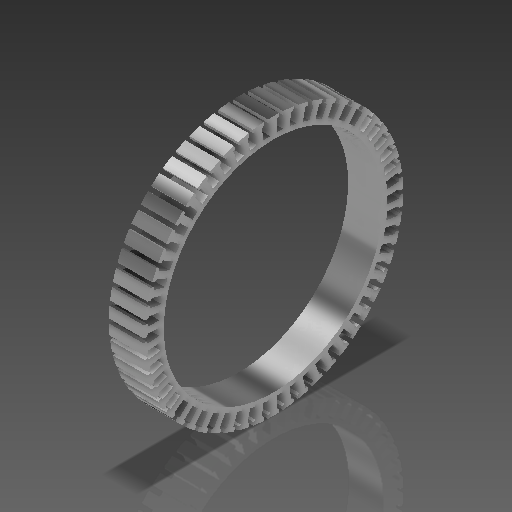
# Autodesk Inventor part: stator
Saved by Autodesk Inventor 2026.2 (Build 302298000, 298)
## iProperties
Created: 2026-05-19
Part Number: stator
Material: Generic
Document SubType Name: Modeling
Designer: LENOVO
Density: 1 g/cm^3
Appearance: Default
Author: LENOVO
Autodesk Inventor part; units mm, degrees
ref_plane "YZ Plane" through (0, 0, 0) normal (1, 0, 0) x (0, 1, 0)
ref_plane "XZ Plane" through (0, 0, 0) normal (0, 1, 0) x (-1, 0, 0)
ref_plane "XY Plane" through (0, 0, 0) normal (0, 0, 1) x (1, 0, 0)
sketch "Sketch1" plane through (0, 0, 0) normal (1, 0, 0) x (0, 1, 0)
  circle A0 centre (0, 0) radius 107.25
  line L0 (127, 0) -> (0, 0) construction
  line L1 (0, 0) -> (127, 0) construction
  line L2 (111.657, -3.1) -> (122.8894, -3.1)
  line L3 (123.8894, -5.3) -> (126.8894, -5.3) construction
  line L4 (123.8894, -5.3) -> (126.8894, -5.3)
  line L5 (111.657, 3.1) -> (122.8894, 3.1)
  line L6 (123.8894, 5.3) -> (126.8894, 5.3) construction
  line L7 (123.8894, 5.3) -> (126.8894, 5.3)
  line L8 (126.8894, -5.3) -> (123.8894, -5.3)
  line L9 (123.8894, -5.3) -> (122.8894, -3.1)
  line L10 (123.8894, 5.3) -> (122.8894, 3.1)
  line L11 (123.667, 9.1185) -> (126.6467, 9.4668) construction
  line L12 (123.667, 9.1185) -> (126.6467, 9.4668)
  line L13 (122.4364, 19.6468) -> (125.4161, 19.9951) construction
  line L14 (122.4364, 19.6468) -> (125.4161, 19.9951)
  line L15 (126.6467, 9.4668) -> (123.667, 9.1185)
  line L16 (123.667, 9.1185) -> (122.4183, 11.1875)
  line L17 (122.4364, 19.6468) -> (121.6985, 17.3456)
  line L18 (111.2619, 9.8835) -> (122.4183, 11.1875)
  line L19 (110.5421, 16.0416) -> (121.6985, 17.3456)
  line L20 (121.7722, 23.4137) -> (124.6913, 24.1056) construction
  line L21 (121.7722, 23.4137) -> (124.6913, 24.1056)
  line L22 (119.3276, 33.728) -> (122.2468, 34.4198) construction
  line L23 (119.3276, 33.728) -> (122.2468, 34.4198)
  line L24 (124.6913, 24.1056) -> (121.7722, 23.4137)
  line L25 (121.7722, 23.4137) -> (120.2918, 25.3238)
  line L26 (119.3276, 33.728) -> (118.862, 31.3567)
  line L27 (109.3622, 22.7334) -> (120.2918, 25.3238)
  line L28 (107.9323, 28.7663) -> (118.862, 31.3567)
  line L29 (118.2306, 37.3923) -> (121.0497, 38.4183) construction
  line L30 (118.2306, 37.3923) -> (121.0497, 38.4183)
  line L31 (114.6052, 47.353) -> (117.4243, 48.3791) construction
  line L32 (114.6052, 47.353) -> (117.4243, 48.3791)
  line L33 (121.0497, 38.4183) -> (118.2306, 37.3923)
  line L34 (118.2306, 37.3923) -> (116.5385, 39.1176)
  line L35 (114.6052, 47.353) -> (114.418, 44.9437)
  line L36 (105.9835, 35.2759) -> (116.5385, 39.1176)
  line L37 (103.863, 41.102) -> (114.418, 44.9437)
  line L38 (113.0902, 50.8652) -> (115.7711, 52.2116) construction
  line L39 (113.0902, 50.8652) -> (115.7711, 52.2116)
  line L40 (108.3329, 60.3377) -> (111.0138, 61.6841) construction
  line L41 (108.3329, 60.3377) -> (111.0138, 61.6841)
  line L42 (115.7711, 52.2116) -> (113.0902, 50.8652)
  line L43 (113.0902, 50.8652) -> (111.2092, 52.3824)
  line L44 (108.3329, 60.3377) -> (108.4267, 57.9229)
  line L45 (101.1716, 47.3413) -> (111.2092, 52.3824)
  line L46 (98.389, 52.8818) -> (108.4267, 57.9229)
  arc A1 (111.657, 3.1) -> (111.2619, 9.8835) centre (0, 0) ccw
  arc A2 (111.2619, -9.8835) -> (111.657, -3.1) centre (0, 0) ccw
  arc A3 (109.3622, -22.7334) -> (110.5421, -16.0416) centre (0, 0) ccw
  arc A4 (105.9835, -35.2759) -> (107.9323, -28.7663) centre (0, 0) ccw
  arc A5 (101.1716, -47.3413) -> (103.863, -41.102) centre (0, 0) ccw
  arc A6 (94.9915, -58.7665) -> (98.389, -52.8818) centre (0, 0) ccw
  arc A7 (87.5268, -69.397) -> (91.5846, -63.9465) centre (0, 0) ccw
  arc A8 (78.8785, -79.089) -> (83.5416, -74.1465) centre (0, 0) ccw
  arc A9 (69.1635, -87.7115) -> (74.3688, -83.3437) centre (0, 0) ccw
  arc A10 (58.5132, -95.1478) -> (64.1903, -91.4138) centre (0, 0) ccw
  arc A11 (47.0715, -101.2974) -> (53.1438, -98.2478) centre (0, 0) ccw
  arc A12 (34.9933, -106.0771) -> (41.3786, -103.7531) centre (0, 0) ccw
  arc A13 (22.4419, -109.4223) -> (29.0538, -107.8553) centre (0, 0) ccw
  arc A14 (9.587, -111.2878) -> (16.3361, -110.499) centre (0, 0) ccw
  arc A15 (-3.3975, -111.6483) -> (3.3975, -111.6483) centre (0, 0) ccw
  arc A16 (-16.3361, -110.499) -> (-9.587, -111.2878) centre (0, 0) ccw
  arc A17 (-29.0538, -107.8553) -> (-22.4419, -109.4223) centre (0, 0) ccw
  arc A18 (-41.3786, -103.7531) -> (-34.9933, -106.0771) centre (0, 0) ccw
  arc A19 (-53.1438, -98.2478) -> (-47.0715, -101.2974) centre (0, 0) ccw
  arc A20 (-64.1903, -91.4138) -> (-58.5132, -95.1478) centre (0, 0) ccw
  arc A21 (-74.3688, -83.3437) -> (-69.1635, -87.7115) centre (0, 0) ccw
  arc A22 (-83.5416, -74.1465) -> (-78.8785, -79.089) centre (0, 0) ccw
  arc A23 (-91.5846, -63.9465) -> (-87.5268, -69.397) centre (0, 0) ccw
  arc A24 (-98.389, -52.8818) -> (-94.9915, -58.7665) centre (0, 0) ccw
  arc A25 (-103.863, -41.102) -> (-101.1716, -47.3413) centre (0, 0) ccw
  arc A26 (-107.9323, -28.7663) -> (-105.9835, -35.2759) centre (0, 0) ccw
  arc A27 (-110.5421, -16.0416) -> (-109.3622, -22.7334) centre (0, 0) ccw
  arc A28 (-111.657, -3.1) -> (-111.2619, -9.8835) centre (0, 0) ccw
  arc A29 (-111.2619, 9.8835) -> (-111.657, 3.1) centre (0, 0) ccw
  arc A30 (-109.3622, 22.7334) -> (-110.5421, 16.0416) centre (0, 0) ccw
  arc A31 (-105.9835, 35.2759) -> (-107.9323, 28.7663) centre (0, 0) ccw
  arc A32 (-101.1716, 47.3413) -> (-103.863, 41.102) centre (0, 0) ccw
  arc A33 (-94.9915, 58.7665) -> (-98.389, 52.8818) centre (0, 0) ccw
  arc A34 (-87.5268, 69.397) -> (-91.5846, 63.9465) centre (0, 0) ccw
  arc A35 (-78.8785, 79.089) -> (-83.5416, 74.1465) centre (0, 0) ccw
  arc A36 (-69.1635, 87.7115) -> (-74.3688, 83.3437) centre (0, 0) ccw
  arc A37 (-58.5132, 95.1478) -> (-64.1903, 91.4138) centre (0, 0) ccw
  arc A38 (-47.0715, 101.2974) -> (-53.1438, 98.2478) centre (0, 0) ccw
  arc A39 (-34.9933, 106.0771) -> (-41.3786, 103.7531) centre (0, 0) ccw
  arc A40 (-22.4419, 109.4223) -> (-29.0538, 107.8553) centre (0, 0) ccw
  arc A41 (-9.587, 111.2878) -> (-16.3361, 110.499) centre (0, 0) ccw
  arc A42 (3.3975, 111.6483) -> (-3.3975, 111.6483) centre (0, 0) ccw
  arc A43 (16.3361, 110.499) -> (9.587, 111.2878) centre (0, 0) ccw
  arc A44 (29.0538, 107.8553) -> (22.4419, 109.4223) centre (0, 0) ccw
  arc A45 (41.3786, 103.7531) -> (34.9933, 106.0771) centre (0, 0) ccw
  arc A46 (53.1438, 98.2478) -> (47.0715, 101.2974) centre (0, 0) ccw
  arc A47 (64.1903, 91.4138) -> (58.5132, 95.1478) centre (0, 0) ccw
  arc A48 (74.3688, 83.3437) -> (69.1635, 87.7115) centre (0, 0) ccw
  arc A49 (83.5416, 74.1465) -> (78.8785, 79.089) centre (0, 0) ccw
  arc A50 (91.5846, 63.9465) -> (87.5268, 69.397) centre (0, 0) ccw
  arc A51 (98.389, 52.8818) -> (94.9915, 58.7665) centre (0, 0) ccw
  arc A52 (107.9323, 28.7663) -> (105.9835, 35.2759) centre (0, 0) ccw
  arc A53 (103.863, 41.102) -> (101.1716, 47.3413) centre (0, 0) ccw
  arc A54 (124.6913, 24.1056) -> (122.2468, 34.4198) centre (0, 0) ccw
  arc A55 (121.0497, 38.4183) -> (117.4243, 48.3791) centre (0, 0) ccw
  arc A56 (115.7711, 52.2116) -> (111.0138, 61.6841) centre (0, 0) ccw
  arc A57 (108.9269, 65.2988) -> (103.1021, 74.1549) centre (0, 0) ccw
  arc A58 (100.6097, 77.5029) -> (93.7961, 85.6229) centre (0, 0) ccw
  arc A59 (90.9318, 88.6589) -> (83.2217, 95.9331) centre (0, 0) ccw
  arc A60 (80.0243, 98.616) -> (71.5218, 104.9458) centre (0, 0) ccw
  arc A61 (68.0346, 107.2394) -> (58.8547, 112.5394) centre (0, 0) ccw
  arc A62 (55.1249, 114.4126) -> (45.3918, 118.6111) centre (0, 0) ccw
  arc A63 (41.4696, 120.0386) -> (31.3149, 123.0787) centre (0, 0) ccw
  arc A64 (27.2536, 124.0413) -> (16.8146, 125.882) centre (0, 0) ccw
  arc A65 (12.669, 126.3665) -> (2.0869, 126.9829) centre (0, 0) ccw
  arc A66 (-2.0869, 126.9829) -> (-12.669, 126.3665) centre (0, 0) ccw
  arc A67 (-16.8146, 125.882) -> (-27.2536, 124.0413) centre (0, 0) ccw
  arc A68 (-31.3149, 123.0787) -> (-41.4696, 120.0386) centre (0, 0) ccw
  arc A69 (-45.3918, 118.6111) -> (-55.1249, 114.4126) centre (0, 0) ccw
  arc A70 (-58.8547, 112.5394) -> (-68.0346, 107.2394) centre (0, 0) ccw
  arc A71 (-71.5218, 104.9458) -> (-80.0243, 98.616) centre (0, 0) ccw
  arc A72 (-83.2217, 95.9331) -> (-90.9318, 88.6589) centre (0, 0) ccw
  arc A73 (-93.7961, 85.6229) -> (-100.6097, 77.5029) centre (0, 0) ccw
  arc A74 (-103.1021, 74.1549) -> (-108.9269, 65.2988) centre (0, 0) ccw
  arc A75 (-111.0138, 61.6841) -> (-115.7711, 52.2116) centre (0, 0) ccw
  arc A76 (-117.4243, 48.3791) -> (-121.0497, 38.4183) centre (0, 0) ccw
  arc A77 (-122.2468, 34.4198) -> (-124.6913, 24.1056) centre (0, 0) ccw
  arc A78 (-125.4161, 19.9951) -> (-126.6467, 9.4668) centre (0, 0) ccw
  arc A79 (-126.8894, 5.3) -> (-126.8894, -5.3) centre (0, 0) ccw
  arc A80 (-126.6467, -9.4668) -> (-125.4161, -19.9951) centre (0, 0) ccw
  arc A81 (-124.6913, -24.1056) -> (-122.2468, -34.4198) centre (0, 0) ccw
  arc A82 (-121.0497, -38.4183) -> (-117.4243, -48.3791) centre (0, 0) ccw
  arc A83 (-115.7711, -52.2116) -> (-111.0138, -61.6841) centre (0, 0) ccw
  arc A84 (-108.9269, -65.2988) -> (-103.1021, -74.1549) centre (0, 0) ccw
  arc A85 (-100.6097, -77.5029) -> (125.4161, 19.9951) centre (0, 0) ccw
  line L47 (106.4204, 63.6502) -> (108.9269, 65.2988) construction
  line L48 (106.4204, 63.6502) -> (108.9269, 65.2988)
  line L49 (100.5957, 72.5064) -> (103.1021, 74.1549) construction
  line L50 (100.5957, 72.5064) -> (103.1021, 74.1549)
  line L51 (108.9269, 65.2988) -> (106.4204, 63.6502)
  line L52 (106.4204, 63.6502) -> (104.376, 64.9388)
  line L53 (100.5957, 72.5064) -> (100.9691, 70.1188)
  line L54 (94.9915, 58.7665) -> (104.376, 64.9388)
  line L55 (91.5846, 63.9465) -> (100.9691, 70.1188)
  line L56 (98.3115, 75.5745) -> (100.6097, 77.5029) construction
  line L57 (98.3115, 75.5745) -> (100.6097, 77.5029)
  line L58 (91.498, 83.6946) -> (93.7961, 85.6229) construction
  line L59 (91.498, 83.6946) -> (93.7961, 85.6229)
  line L60 (100.6097, 77.5029) -> (98.3115, 75.5745)
  line L61 (98.3115, 75.5745) -> (96.1314, 76.617)
  line L62 (91.498, 83.6946) -> (92.1461, 81.3665)
  line L63 (87.5268, 69.397) -> (96.1314, 76.617)
  line L64 (83.5416, 74.1465) -> (92.1461, 81.3665)
  line L65 (88.8731, 86.4768) -> (90.9318, 88.6589) construction
  line L66 (88.8731, 86.4768) -> (90.9318, 88.6589)
  line L67 (81.163, 93.7509) -> (83.2217, 95.9331) construction
  line L68 (81.163, 93.7509) -> (83.2217, 95.9331)
  line L69 (90.9318, 88.6589) -> (88.8731, 86.4768)
  line L70 (88.8731, 86.4768) -> (86.5867, 87.2591)
  line L71 (81.163, 93.7509) -> (82.0769, 91.5138)
  line L72 (78.8785, 79.089) -> (86.5867, 87.2591)
  line L73 (74.3688, 83.3437) -> (82.0769, 91.5138)
  line L74 (78.2328, 96.2096) -> (80.0243, 98.616) construction
  line L75 (78.2328, 96.2096) -> (80.0243, 98.616)
  line L76 (69.7303, 102.5395) -> (71.5218, 104.9458) construction
  line L77 (69.7303, 102.5395) -> (71.5218, 104.9458)
  line L78 (80.0243, 98.616) -> (78.2328, 96.2096)
  line L79 (78.2328, 96.2096) -> (75.871, 96.7212)
  line L80 (69.7303, 102.5395) -> (70.8979, 100.4236)
  line L81 (69.1635, 87.7115) -> (75.871, 96.7212)
  line L82 (64.1903, 91.4138) -> (70.8979, 100.4236)
  line L83 (66.5346, 104.6413) -> (68.0346, 107.2394) construction
  line L84 (66.5346, 104.6413) -> (68.0346, 107.2394)
  line L85 (57.3547, 109.9413) -> (58.8547, 112.5394) construction
  line L86 (57.3547, 109.9413) -> (58.8547, 112.5394)
  line L87 (68.0346, 107.2394) -> (66.5346, 104.6413)
  line L88 (66.5346, 104.6413) -> (64.1294, 104.8753)
  line L89 (57.3547, 109.9413) -> (58.76, 107.9753)
  line L90 (58.5132, 95.1478) -> (64.1294, 104.8753)
  line L91 (53.1438, 98.2478) -> (58.76, 107.9753)
  line L92 (53.9366, 111.658) -> (55.1249, 114.4126) construction
  line L93 (53.9366, 111.658) -> (55.1249, 114.4126)
  line L94 (44.2035, 115.8564) -> (45.3918, 118.6111) construction
  line L95 (44.2035, 115.8564) -> (45.3918, 118.6111)
  line L96 (55.1249, 114.4126) -> (53.9366, 111.658)
  line L97 (53.9366, 111.658) -> (51.5205, 111.6111)
  line L98 (44.2035, 115.8564) -> (45.8275, 114.0668)
  line L99 (47.0715, 101.2974) -> (51.5205, 111.6111)
  line L100 (41.3786, 103.7531) -> (45.8275, 114.0668)
  line L101 (40.6092, 117.1647) -> (41.4696, 120.0386) construction
  line L102 (40.6092, 117.1647) -> (41.4696, 120.0386)
  line L103 (30.4545, 120.2048) -> (31.3149, 123.0787) construction
  line L104 (30.4545, 120.2048) -> (31.3149, 123.0787)
  line L105 (41.4696, 120.0386) -> (40.6092, 117.1647)
  line L106 (40.6092, 117.1647) -> (38.2148, 116.8376)
  line L107 (30.4545, 120.2048) -> (32.2753, 118.6158)
  line L108 (34.9933, 106.0771) -> (38.2148, 116.8376)
  line L109 (29.0538, 107.8553) -> (32.2753, 118.6158)
  line L110 (26.7326, 121.0869) -> (27.2536, 124.0413) construction
  line L111 (26.7326, 121.0869) -> (27.2536, 124.0413)
  line L112 (16.2937, 122.9275) -> (16.8146, 125.882) construction
  line L113 (16.2937, 122.9275) -> (16.8146, 125.882)
  line L114 (27.2536, 124.0413) -> (26.7326, 121.0869)
  line L115 (26.7326, 121.0869) -> (24.3924, 120.4841)
  line L116 (16.2937, 122.9275) -> (18.2866, 121.5607)
  line L117 (22.4419, 109.4223) -> (24.3924, 120.4841)
  line L118 (16.3361, 110.499) -> (18.2866, 121.5607)
  line L119 (12.4946, 123.3716) -> (12.669, 126.3665) construction
  line L120 (12.4946, 123.3716) -> (12.669, 126.3665)
  line L121 (1.9125, 123.9879) -> (2.0869, 126.9829) construction
  line L122 (1.9125, 123.9879) -> (2.0869, 126.9829)
  line L123 (12.669, 126.3665) -> (12.4946, 123.3716)
  line L124 (12.4946, 123.3716) -> (10.2401, 122.5012)
  line L125 (1.9125, 123.9879) -> (4.0506, 122.8617)
  line L126 (9.587, 111.2878) -> (10.2401, 122.5012)
  line L127 (3.3975, 111.6483) -> (4.0506, 122.8617)
  line L128 (-1.9125, 123.9879) -> (-2.0869, 126.9829) construction
  line L129 (-1.9125, 123.9879) -> (-2.0869, 126.9829)
  line L130 (-12.4946, 123.3716) -> (-12.669, 126.3665) construction
  line L131 (-12.4946, 123.3716) -> (-12.669, 126.3665)
  line L132 (-2.0869, 126.9829) -> (-1.9125, 123.9879)
  line L133 (-1.9125, 123.9879) -> (-4.0506, 122.8617)
  line L134 (-12.4946, 123.3716) -> (-10.2401, 122.5012)
  line L135 (-3.3975, 111.6483) -> (-4.0506, 122.8617)
  line L136 (-9.587, 111.2878) -> (-10.2401, 122.5012)
  line L137 (-16.2937, 122.9275) -> (-16.8146, 125.882) construction
  line L138 (-16.2937, 122.9275) -> (-16.8146, 125.882)
  line L139 (-26.7326, 121.0869) -> (-27.2536, 124.0413) construction
  line L140 (-26.7326, 121.0869) -> (-27.2536, 124.0413)
  line L141 (-16.8146, 125.882) -> (-16.2937, 122.9275)
  line L142 (-16.2937, 122.9275) -> (-18.2866, 121.5607)
  line L143 (-26.7326, 121.0869) -> (-24.3924, 120.4841)
  line L144 (-16.3361, 110.499) -> (-18.2866, 121.5607)
  line L145 (-22.4419, 109.4223) -> (-24.3924, 120.4841)
  line L146 (-30.4545, 120.2048) -> (-31.3149, 123.0787) construction
  line L147 (-30.4545, 120.2048) -> (-31.3149, 123.0787)
  line L148 (-40.6092, 117.1647) -> (-41.4696, 120.0386) construction
  line L149 (-40.6092, 117.1647) -> (-41.4696, 120.0386)
  line L150 (-31.3149, 123.0787) -> (-30.4545, 120.2048)
  line L151 (-30.4545, 120.2048) -> (-32.2753, 118.6158)
  line L152 (-40.6092, 117.1647) -> (-38.2148, 116.8376)
  line L153 (-29.0538, 107.8553) -> (-32.2753, 118.6158)
  line L154 (-34.9933, 106.0771) -> (-38.2148, 116.8376)
  line L155 (-44.2035, 115.8564) -> (-45.3918, 118.6111) construction
  line L156 (-44.2035, 115.8564) -> (-45.3918, 118.6111)
  line L157 (-53.9366, 111.658) -> (-55.1249, 114.4126) construction
  line L158 (-53.9366, 111.658) -> (-55.1249, 114.4126)
  line L159 (-45.3918, 118.6111) -> (-44.2035, 115.8564)
  line L160 (-44.2035, 115.8564) -> (-45.8275, 114.0668)
  line L161 (-53.9366, 111.658) -> (-51.5205, 111.6111)
  line L162 (-41.3786, 103.7531) -> (-45.8275, 114.0668)
  line L163 (-47.0715, 101.2974) -> (-51.5205, 111.6111)
  line L164 (-57.3547, 109.9413) -> (-58.8547, 112.5394) construction
  line L165 (-57.3547, 109.9413) -> (-58.8547, 112.5394)
  line L166 (-66.5346, 104.6413) -> (-68.0346, 107.2394) construction
  line L167 (-66.5346, 104.6413) -> (-68.0346, 107.2394)
  line L168 (-58.8547, 112.5394) -> (-57.3547, 109.9413)
  line L169 (-57.3547, 109.9413) -> (-58.76, 107.9753)
  line L170 (-66.5346, 104.6413) -> (-64.1294, 104.8753)
  line L171 (-53.1438, 98.2478) -> (-58.76, 107.9753)
  line L172 (-58.5132, 95.1478) -> (-64.1294, 104.8753)
  line L173 (-69.7303, 102.5395) -> (-71.5218, 104.9458) construction
  line L174 (-69.7303, 102.5395) -> (-71.5218, 104.9458)
  line L175 (-78.2328, 96.2096) -> (-80.0243, 98.616) construction
  line L176 (-78.2328, 96.2096) -> (-80.0243, 98.616)
  line L177 (-71.5218, 104.9458) -> (-69.7303, 102.5395)
  line L178 (-69.7303, 102.5395) -> (-70.8979, 100.4236)
  line L179 (-78.2328, 96.2096) -> (-75.871, 96.7212)
  line L180 (-64.1903, 91.4138) -> (-70.8979, 100.4236)
  line L181 (-69.1635, 87.7115) -> (-75.871, 96.7212)
  line L182 (-81.163, 93.7509) -> (-83.2217, 95.9331) construction
  line L183 (-81.163, 93.7509) -> (-83.2217, 95.9331)
  line L184 (-88.8731, 86.4768) -> (-90.9318, 88.6589) construction
  line L185 (-88.8731, 86.4768) -> (-90.9318, 88.6589)
  line L186 (-83.2217, 95.9331) -> (-81.163, 93.7509)
  line L187 (-81.163, 93.7509) -> (-82.0769, 91.5138)
  line L188 (-88.8731, 86.4768) -> (-86.5867, 87.2591)
  line L189 (-74.3688, 83.3437) -> (-82.0769, 91.5138)
  line L190 (-78.8785, 79.089) -> (-86.5867, 87.2591)
  line L191 (-91.498, 83.6946) -> (-93.7961, 85.6229) construction
  line L192 (-91.498, 83.6946) -> (-93.7961, 85.6229)
  line L193 (-98.3115, 75.5745) -> (-100.6097, 77.5029) construction
  line L194 (-98.3115, 75.5745) -> (-100.6097, 77.5029)
  line L195 (-93.7961, 85.6229) -> (-91.498, 83.6946)
  line L196 (-91.498, 83.6946) -> (-92.1461, 81.3665)
  line L197 (-98.3115, 75.5745) -> (-96.1314, 76.617)
  line L198 (-83.5416, 74.1465) -> (-92.1461, 81.3665)
  line L199 (-87.5268, 69.397) -> (-96.1314, 76.617)
  line L200 (-100.5957, 72.5064) -> (-103.1021, 74.1549) construction
  line L201 (-100.5957, 72.5064) -> (-103.1021, 74.1549)
  line L202 (-106.4204, 63.6502) -> (-108.9269, 65.2988) construction
  line L203 (-106.4204, 63.6502) -> (-108.9269, 65.2988)
  line L204 (-103.1021, 74.1549) -> (-100.5957, 72.5064)
  line L205 (-100.5957, 72.5064) -> (-100.9691, 70.1188)
  line L206 (-106.4204, 63.6502) -> (-104.376, 64.9388)
  line L207 (-91.5846, 63.9465) -> (-100.9691, 70.1188)
  line L208 (-94.9915, 58.7665) -> (-104.376, 64.9388)
  line L209 (-108.3329, 60.3377) -> (-111.0138, 61.6841) construction
  line L210 (-108.3329, 60.3377) -> (-111.0138, 61.6841)
  line L211 (-113.0902, 50.8652) -> (-115.7711, 52.2116) construction
  line L212 (-113.0902, 50.8652) -> (-115.7711, 52.2116)
  line L213 (-111.0138, 61.6841) -> (-108.3329, 60.3377)
  line L214 (-108.3329, 60.3377) -> (-108.4267, 57.9229)
  line L215 (-113.0902, 50.8652) -> (-111.2092, 52.3824)
  line L216 (-98.389, 52.8818) -> (-108.4267, 57.9229)
  line L217 (-101.1716, 47.3413) -> (-111.2092, 52.3824)
  line L218 (-114.6052, 47.353) -> (-117.4243, 48.3791) construction
  line L219 (-114.6052, 47.353) -> (-117.4243, 48.3791)
  line L220 (-118.2306, 37.3923) -> (-121.0497, 38.4183) construction
  line L221 (-118.2306, 37.3923) -> (-121.0497, 38.4183)
  line L222 (-117.4243, 48.3791) -> (-114.6052, 47.353)
  line L223 (-114.6052, 47.353) -> (-114.418, 44.9437)
  line L224 (-118.2306, 37.3923) -> (-116.5385, 39.1176)
  line L225 (-103.863, 41.102) -> (-114.418, 44.9437)
  line L226 (-105.9835, 35.2759) -> (-116.5385, 39.1176)
  line L227 (-119.3276, 33.728) -> (-122.2468, 34.4198) construction
  line L228 (-119.3276, 33.728) -> (-122.2468, 34.4198)
  line L229 (-121.7722, 23.4137) -> (-124.6913, 24.1056) construction
  line L230 (-121.7722, 23.4137) -> (-124.6913, 24.1056)
  line L231 (-122.2468, 34.4198) -> (-119.3276, 33.728)
  line L232 (-119.3276, 33.728) -> (-118.862, 31.3567)
  line L233 (-121.7722, 23.4137) -> (-120.2918, 25.3238)
  line L234 (-107.9323, 28.7663) -> (-118.862, 31.3567)
  line L235 (-109.3622, 22.7334) -> (-120.2918, 25.3238)
  line L236 (-122.4364, 19.6468) -> (-125.4161, 19.9951) construction
  line L237 (-122.4364, 19.6468) -> (-125.4161, 19.9951)
  line L238 (-123.667, 9.1185) -> (-126.6467, 9.4668) construction
  line L239 (-123.667, 9.1185) -> (-126.6467, 9.4668)
  line L240 (-125.4161, 19.9951) -> (-122.4364, 19.6468)
  line L241 (-122.4364, 19.6468) -> (-121.6985, 17.3456)
  line L242 (-123.667, 9.1185) -> (-122.4183, 11.1875)
  line L243 (-110.5421, 16.0416) -> (-121.6985, 17.3456)
  line L244 (-111.2619, 9.8835) -> (-122.4183, 11.1875)
  line L245 (-123.8894, 5.3) -> (-126.8894, 5.3) construction
  line L246 (-123.8894, 5.3) -> (-126.8894, 5.3)
  line L247 (-123.8894, -5.3) -> (-126.8894, -5.3) construction
  line L248 (-123.8894, -5.3) -> (-126.8894, -5.3)
  line L249 (-126.8894, 5.3) -> (-123.8894, 5.3)
  line L250 (-123.8894, 5.3) -> (-122.8894, 3.1)
  line L251 (-123.8894, -5.3) -> (-122.8894, -3.1)
  line L252 (-111.657, 3.1) -> (-122.8894, 3.1)
  line L253 (-111.657, -3.1) -> (-122.8894, -3.1)
  line L254 (-123.667, -9.1185) -> (-126.6467, -9.4668) construction
  line L255 (-123.667, -9.1185) -> (-126.6467, -9.4668)
  line L256 (-122.4364, -19.6468) -> (-125.4161, -19.9951) construction
  line L257 (-122.4364, -19.6468) -> (-125.4161, -19.9951)
  line L258 (-126.6467, -9.4668) -> (-123.667, -9.1185)
  line L259 (-123.667, -9.1185) -> (-122.4183, -11.1875)
  line L260 (-122.4364, -19.6468) -> (-121.6985, -17.3456)
  line L261 (-111.2619, -9.8835) -> (-122.4183, -11.1875)
  line L262 (-110.5421, -16.0416) -> (-121.6985, -17.3456)
  line L263 (-121.7722, -23.4137) -> (-124.6913, -24.1056) construction
  line L264 (-121.7722, -23.4137) -> (-124.6913, -24.1056)
  line L265 (-119.3276, -33.728) -> (-122.2468, -34.4198) construction
  line L266 (-119.3276, -33.728) -> (-122.2468, -34.4198)
  line L267 (-124.6913, -24.1056) -> (-121.7722, -23.4137)
  line L268 (-121.7722, -23.4137) -> (-120.2918, -25.3238)
  line L269 (-119.3276, -33.728) -> (-118.862, -31.3567)
  line L270 (-109.3622, -22.7334) -> (-120.2918, -25.3238)
  line L271 (-107.9323, -28.7663) -> (-118.862, -31.3567)
  line L272 (-118.2306, -37.3923) -> (-121.0497, -38.4183) construction
  line L273 (-118.2306, -37.3923) -> (-121.0497, -38.4183)
  line L274 (-114.6052, -47.353) -> (-117.4243, -48.3791) construction
  line L275 (-114.6052, -47.353) -> (-117.4243, -48.3791)
  line L276 (-121.0497, -38.4183) -> (-118.2306, -37.3923)
  line L277 (-118.2306, -37.3923) -> (-116.5385, -39.1176)
  line L278 (-114.6052, -47.353) -> (-114.418, -44.9437)
  line L279 (-105.9835, -35.2759) -> (-116.5385, -39.1176)
  line L280 (-103.863, -41.102) -> (-114.418, -44.9437)
  line L281 (-113.0902, -50.8652) -> (-115.7711, -52.2116) construction
  line L282 (-113.0902, -50.8652) -> (-115.7711, -52.2116)
  line L283 (-108.3329, -60.3377) -> (-111.0138, -61.6841) construction
  line L284 (-108.3329, -60.3377) -> (-111.0138, -61.6841)
  line L285 (-115.7711, -52.2116) -> (-113.0902, -50.8652)
  line L286 (-113.0902, -50.8652) -> (-111.2092, -52.3824)
  line L287 (-108.3329, -60.3377) -> (-108.4267, -57.9229)
  line L288 (-101.1716, -47.3413) -> (-111.2092, -52.3824)
  line L289 (-98.389, -52.8818) -> (-108.4267, -57.9229)
  line L290 (-106.4204, -63.6502) -> (-108.9269, -65.2988) construction
  line L291 (-106.4204, -63.6502) -> (-108.9269, -65.2988)
  line L292 (-100.5957, -72.5064) -> (-103.1021, -74.1549) construction
  line L293 (-100.5957, -72.5064) -> (-103.1021, -74.1549)
  line L294 (-108.9269, -65.2988) -> (-106.4204, -63.6502)
  line L295 (-106.4204, -63.6502) -> (-104.376, -64.9388)
  line L296 (-100.5957, -72.5064) -> (-100.9691, -70.1188)
  line L297 (-94.9915, -58.7665) -> (-104.376, -64.9388)
  line L298 (-91.5846, -63.9465) -> (-100.9691, -70.1188)
  line L299 (-98.3115, -75.5745) -> (-100.6097, -77.5029) construction
  line L300 (-98.3115, -75.5745) -> (-100.6097, -77.5029)
  line L301 (-91.498, -83.6946) -> (-93.7961, -85.6229) construction
  line L302 (-91.498, -83.6946) -> (-93.7961, -85.6229)
  line L303 (-100.6097, -77.5029) -> (-98.3115, -75.5745)
  line L304 (-98.3115, -75.5745) -> (-96.1314, -76.617)
  line L305 (-91.498, -83.6946) -> (-92.1461, -81.3665)
  line L306 (-87.5268, -69.397) -> (-96.1314, -76.617)
  line L307 (-83.5416, -74.1465) -> (-92.1461, -81.3665)
  line L308 (-88.8731, -86.4768) -> (-90.9318, -88.6589) construction
  line L309 (-88.8731, -86.4768) -> (-90.9318, -88.6589)
  line L310 (-81.163, -93.7509) -> (-83.2217, -95.9331) construction
  line L311 (-81.163, -93.7509) -> (-83.2217, -95.9331)
  line L312 (-90.9318, -88.6589) -> (-88.8731, -86.4768)
  line L313 (-88.8731, -86.4768) -> (-86.5867, -87.2591)
  line L314 (-81.163, -93.7509) -> (-82.0769, -91.5138)
  line L315 (-78.8785, -79.089) -> (-86.5867, -87.2591)
  line L316 (-74.3688, -83.3437) -> (-82.0769, -91.5138)
  line L317 (-78.2328, -96.2096) -> (-80.0243, -98.616) construction
  line L318 (-78.2328, -96.2096) -> (-80.0243, -98.616)
  line L319 (-69.7303, -102.5395) -> (-71.5218, -104.9458) construction
  line L320 (-69.7303, -102.5395) -> (-71.5218, -104.9458)
  line L321 (-80.0243, -98.616) -> (-78.2328, -96.2096)
  line L322 (-78.2328, -96.2096) -> (-75.871, -96.7212)
  line L323 (-69.7303, -102.5395) -> (-70.8979, -100.4236)
  line L324 (-69.1635, -87.7115) -> (-75.871, -96.7212)
  line L325 (-64.1903, -91.4138) -> (-70.8979, -100.4236)
  line L326 (-66.5346, -104.6413) -> (-68.0346, -107.2394) construction
  line L327 (-66.5346, -104.6413) -> (-68.0346, -107.2394)
  line L328 (-57.3547, -109.9413) -> (-58.8547, -112.5394) construction
  line L329 (-57.3547, -109.9413) -> (-58.8547, -112.5394)
  line L330 (-68.0346, -107.2394) -> (-66.5346, -104.6413)
  line L331 (-66.5346, -104.6413) -> (-64.1294, -104.8753)
  line L332 (-57.3547, -109.9413) -> (-58.76, -107.9753)
  line L333 (-58.5132, -95.1478) -> (-64.1294, -104.8753)
  line L334 (-53.1438, -98.2478) -> (-58.76, -107.9753)
  line L335 (-53.9366, -111.658) -> (-55.1249, -114.4126) construction
  line L336 (-53.9366, -111.658) -> (-55.1249, -114.4126)
  line L337 (-44.2035, -115.8564) -> (-45.3918, -118.6111) construction
  line L338 (-44.2035, -115.8564) -> (-45.3918, -118.6111)
  line L339 (-55.1249, -114.4126) -> (-53.9366, -111.658)
  line L340 (-53.9366, -111.658) -> (-51.5205, -111.6111)
  line L341 (-44.2035, -115.8564) -> (-45.8275, -114.0668)
  line L342 (-47.0715, -101.2974) -> (-51.5205, -111.6111)
  line L343 (-41.3786, -103.7531) -> (-45.8275, -114.0668)
  line L344 (-40.6092, -117.1647) -> (-41.4696, -120.0386) construction
  line L345 (-40.6092, -117.1647) -> (-41.4696, -120.0386)
  line L346 (-30.4545, -120.2048) -> (-31.3149, -123.0787) construction
  line L347 (-30.4545, -120.2048) -> (-31.3149, -123.0787)
  line L348 (-41.4696, -120.0386) -> (-40.6092, -117.1647)
  line L349 (-40.6092, -117.1647) -> (-38.2148, -116.8376)
  line L350 (-30.4545, -120.2048) -> (-32.2753, -118.6158)
  line L351 (-34.9933, -106.0771) -> (-38.2148, -116.8376)
  line L352 (-29.0538, -107.8553) -> (-32.2753, -118.6158)
  line L353 (-26.7326, -121.0869) -> (-27.2536, -124.0413) construction
  line L354 (-26.7326, -121.0869) -> (-27.2536, -124.0413)
  line L355 (-16.2937, -122.9275) -> (-16.8146, -125.882) construction
  line L356 (-16.2937, -122.9275) -> (-16.8146, -125.882)
  line L357 (-27.2536, -124.0413) -> (-26.7326, -121.0869)
  line L358 (-26.7326, -121.0869) -> (-24.3924, -120.4841)
  line L359 (-16.2937, -122.9275) -> (-18.2866, -121.5607)
  line L360 (-22.4419, -109.4223) -> (-24.3924, -120.4841)
  line L361 (-16.3361, -110.499) -> (-18.2866, -121.5607)
  line L362 (-12.4946, -123.3716) -> (-12.669, -126.3665) construction
  line L363 (-12.4946, -123.3716) -> (-12.669, -126.3665)
  line L364 (-1.9125, -123.9879) -> (-2.0869, -126.9829) construction
  line L365 (-1.9125, -123.9879) -> (-2.0869, -126.9829)
  line L366 (-12.669, -126.3665) -> (-12.4946, -123.3716)
  line L367 (-12.4946, -123.3716) -> (-10.2401, -122.5012)
  line L368 (-1.9125, -123.9879) -> (-4.0506, -122.8617)
  line L369 (-9.587, -111.2878) -> (-10.2401, -122.5012)
  line L370 (-3.3975, -111.6483) -> (-4.0506, -122.8617)
  line L371 (1.9125, -123.9879) -> (2.0869, -126.9829) construction
  line L372 (1.9125, -123.9879) -> (2.0869, -126.9829)
  line L373 (12.4946, -123.3716) -> (12.669, -126.3665) construction
  line L374 (12.4946, -123.3716) -> (12.669, -126.3665)
  line L375 (2.0869, -126.9829) -> (1.9125, -123.9879)
  line L376 (1.9125, -123.9879) -> (4.0506, -122.8617)
  line L377 (12.4946, -123.3716) -> (10.2401, -122.5012)
  line L378 (3.3975, -111.6483) -> (4.0506, -122.8617)
  line L379 (9.587, -111.2878) -> (10.2401, -122.5012)
  line L380 (16.2937, -122.9275) -> (16.8146, -125.882) construction
  line L381 (16.2937, -122.9275) -> (16.8146, -125.882)
  line L382 (26.7326, -121.0869) -> (27.2536, -124.0413) construction
  line L383 (26.7326, -121.0869) -> (27.2536, -124.0413)
  line L384 (16.8146, -125.882) -> (16.2937, -122.9275)
  line L385 (16.2937, -122.9275) -> (18.2866, -121.5607)
  line L386 (26.7326, -121.0869) -> (24.3924, -120.4841)
  line L387 (16.3361, -110.499) -> (18.2866, -121.5607)
  line L388 (22.4419, -109.4223) -> (24.3924, -120.4841)
  line L389 (30.4545, -120.2048) -> (31.3149, -123.0787) construction
  line L390 (30.4545, -120.2048) -> (31.3149, -123.0787)
  line L391 (40.6092, -117.1647) -> (41.4696, -120.0386) construction
  line L392 (40.6092, -117.1647) -> (41.4696, -120.0386)
  line L393 (31.3149, -123.0787) -> (30.4545, -120.2048)
  line L394 (30.4545, -120.2048) -> (32.2753, -118.6158)
  line L395 (40.6092, -117.1647) -> (38.2148, -116.8376)
  line L396 (29.0538, -107.8553) -> (32.2753, -118.6158)
  line L397 (34.9933, -106.0771) -> (38.2148, -116.8376)
  line L398 (44.2035, -115.8564) -> (45.3918, -118.6111) construction
  line L399 (44.2035, -115.8564) -> (45.3918, -118.6111)
  line L400 (53.9366, -111.658) -> (55.1249, -114.4126) construction
  line L401 (53.9366, -111.658) -> (55.1249, -114.4126)
  line L402 (45.3918, -118.6111) -> (44.2035, -115.8564)
  line L403 (44.2035, -115.8564) -> (45.8275, -114.0668)
  line L404 (53.9366, -111.658) -> (51.5205, -111.6111)
  line L405 (41.3786, -103.7531) -> (45.8275, -114.0668)
  line L406 (47.0715, -101.2974) -> (51.5205, -111.6111)
  line L407 (57.3547, -109.9413) -> (58.8547, -112.5394) construction
  line L408 (57.3547, -109.9413) -> (58.8547, -112.5394)
  line L409 (66.5346, -104.6413) -> (68.0346, -107.2394) construction
  line L410 (66.5346, -104.6413) -> (68.0346, -107.2394)
  line L411 (58.8547, -112.5394) -> (57.3547, -109.9413)
  line L412 (57.3547, -109.9413) -> (58.76, -107.9753)
  line L413 (66.5346, -104.6413) -> (64.1294, -104.8753)
  line L414 (53.1438, -98.2478) -> (58.76, -107.9753)
  line L415 (58.5132, -95.1478) -> (64.1294, -104.8753)
  line L416 (69.7303, -102.5395) -> (71.5218, -104.9458) construction
  line L417 (69.7303, -102.5395) -> (71.5218, -104.9458)
  line L418 (78.2328, -96.2096) -> (80.0243, -98.616) construction
  line L419 (78.2328, -96.2096) -> (80.0243, -98.616)
  line L420 (71.5218, -104.9458) -> (69.7303, -102.5395)
  line L421 (69.7303, -102.5395) -> (70.8979, -100.4236)
  line L422 (78.2328, -96.2096) -> (75.871, -96.7212)
  line L423 (64.1903, -91.4138) -> (70.8979, -100.4236)
  line L424 (69.1635, -87.7115) -> (75.871, -96.7212)
  line L425 (81.163, -93.7509) -> (83.2217, -95.9331) construction
  line L426 (81.163, -93.7509) -> (83.2217, -95.9331)
  line L427 (88.8731, -86.4768) -> (90.9318, -88.6589) construction
  line L428 (88.8731, -86.4768) -> (90.9318, -88.6589)
  line L429 (83.2217, -95.9331) -> (81.163, -93.7509)
  line L430 (81.163, -93.7509) -> (82.0769, -91.5138)
  line L431 (88.8731, -86.4768) -> (86.5867, -87.2591)
  line L432 (74.3688, -83.3437) -> (82.0769, -91.5138)
  line L433 (78.8785, -79.089) -> (86.5867, -87.2591)
  line L434 (91.498, -83.6946) -> (93.7961, -85.6229) construction
  line L435 (91.498, -83.6946) -> (93.7961, -85.6229)
  line L436 (98.3115, -75.5745) -> (100.6097, -77.5029) construction
  line L437 (98.3115, -75.5745) -> (100.6097, -77.5029)
  line L438 (93.7961, -85.6229) -> (91.498, -83.6946)
  line L439 (91.498, -83.6946) -> (92.1461, -81.3665)
  line L440 (98.3115, -75.5745) -> (96.1314, -76.617)
  line L441 (83.5416, -74.1465) -> (92.1461, -81.3665)
  line L442 (87.5268, -69.397) -> (96.1314, -76.617)
  line L443 (100.5957, -72.5064) -> (103.1021, -74.1549) construction
  line L444 (100.5957, -72.5064) -> (103.1021, -74.1549)
  line L445 (106.4204, -63.6502) -> (108.9269, -65.2988) construction
  line L446 (106.4204, -63.6502) -> (108.9269, -65.2988)
  line L447 (103.1021, -74.1549) -> (100.5957, -72.5064)
  line L448 (100.5957, -72.5064) -> (100.9691, -70.1188)
  line L449 (106.4204, -63.6502) -> (104.376, -64.9388)
  line L450 (91.5846, -63.9465) -> (100.9691, -70.1188)
  line L451 (94.9915, -58.7665) -> (104.376, -64.9388)
  line L452 (108.3329, -60.3377) -> (111.0138, -61.6841) construction
  line L453 (108.3329, -60.3377) -> (111.0138, -61.6841)
  line L454 (113.0902, -50.8652) -> (115.7711, -52.2116) construction
  line L455 (113.0902, -50.8652) -> (115.7711, -52.2116)
  line L456 (111.0138, -61.6841) -> (108.3329, -60.3377)
  line L457 (108.3329, -60.3377) -> (108.4267, -57.9229)
  line L458 (113.0902, -50.8652) -> (111.2092, -52.3824)
  line L459 (98.389, -52.8818) -> (108.4267, -57.9229)
  line L460 (101.1716, -47.3413) -> (111.2092, -52.3824)
  line L461 (114.6052, -47.353) -> (117.4243, -48.3791) construction
  line L462 (114.6052, -47.353) -> (117.4243, -48.3791)
  line L463 (118.2306, -37.3923) -> (121.0497, -38.4183) construction
  line L464 (118.2306, -37.3923) -> (121.0497, -38.4183)
  line L465 (117.4243, -48.3791) -> (114.6052, -47.353)
  line L466 (114.6052, -47.353) -> (114.418, -44.9437)
  line L467 (118.2306, -37.3923) -> (116.5385, -39.1176)
  line L468 (103.863, -41.102) -> (114.418, -44.9437)
  line L469 (105.9835, -35.2759) -> (116.5385, -39.1176)
  line L470 (119.3276, -33.728) -> (122.2468, -34.4198) construction
  line L471 (119.3276, -33.728) -> (122.2468, -34.4198)
  line L472 (121.7722, -23.4137) -> (124.6913, -24.1056) construction
  line L473 (121.7722, -23.4137) -> (124.6913, -24.1056)
  line L474 (122.2468, -34.4198) -> (119.3276, -33.728)
  line L475 (119.3276, -33.728) -> (118.862, -31.3567)
  line L476 (121.7722, -23.4137) -> (120.2918, -25.3238)
  line L477 (107.9323, -28.7663) -> (118.862, -31.3567)
  line L478 (109.3622, -22.7334) -> (120.2918, -25.3238)
  line L479 (122.4364, -19.6468) -> (125.4161, -19.9951) construction
  line L480 (122.4364, -19.6468) -> (125.4161, -19.9951)
  line L481 (123.667, -9.1185) -> (126.6467, -9.4668) construction
  line L482 (123.667, -9.1185) -> (126.6467, -9.4668)
  line L483 (125.4161, -19.9951) -> (122.4364, -19.6468)
  line L484 (122.4364, -19.6468) -> (121.6985, -17.3456)
  line L485 (123.667, -9.1185) -> (122.4183, -11.1875)
  line L486 (110.5421, -16.0416) -> (121.6985, -17.3456)
  line L487 (111.2619, -9.8835) -> (122.4183, -11.1875)
  circle A86 centre (0, 0) radius 111.7
  circle A87 centre (0, 0) radius 127
  point P0 (122.8894, -5.3)
  point P1 (122.8894, 5.3)
  point P2 (126.1413, 14.7438)
  point P3 (122.6737, 9.0024)
  point P4 (121.4431, 19.5307)
  point P5 (123.5767, 29.2882)
  point P6 (120.7991, 23.1831)
  point P7 (118.3546, 33.4974)
  point P8 (119.341, 43.4366)
  point P9 (117.2909, 37.0503)
  point P10 (113.6655, 47.011)
  point P11 (113.4913, 56.9975)
  point P12 (112.1966, 50.4164)
  point P13 (107.4393, 59.8889)
  point P14 (106.107, 69.7876)
  point P15 (105.585, 63.1007)
  point P16 (99.7602, 71.9569)
  point P17 (97.2876, 81.634)
  point P18 (97.5455, 74.9317)
  point P19 (90.7319, 83.0518)
  point P20 (87.1527, 92.3765)
  point P21 (88.1869, 85.7494)
  point P22 (80.4767, 93.0236)
  point P23 (75.8391, 101.8696)
  point P24 (77.6357, 95.4075)
  point P25 (69.1332, 101.7373)
  point P26 (63.5, 109.9852)
  point P27 (66.0346, 103.7753)
  point P28 (56.8547, 109.0753)
  point P29 (50.3021, 116.6134)
  point P30 (53.5405, 110.7398)
  point P31 (43.8074, 114.9382)
  point P32 (36.424, 121.6647)
  point P33 (40.3224, 116.2067)
  point P34 (30.1677, 119.2468)
  point P35 (22.0533, 125.0706)
  point P36 (26.559, 120.1021)
  point P37 (16.12, 121.9427)
  point P38 (7.3844, 126.7851)
  point P39 (12.4364, 122.3733)
  point P40 (1.8543, 122.9896)
  point P41 (-7.3844, 126.7851)
  point P42 (-1.8543, 122.9896)
  point P43 (-12.4364, 122.3733)
  point P44 (-22.0533, 125.0706)
  point P45 (-16.12, 121.9427)
  point P46 (-26.559, 120.1021)
  point P47 (-36.424, 121.6647)
  point P48 (-30.1677, 119.2468)
  point P49 (-40.3224, 116.2067)
  point P50 (-50.3021, 116.6134)
  point P51 (-43.8074, 114.9382)
  point P52 (-53.5405, 110.7398)
  point P53 (-63.5, 109.9852)
  point P54 (-56.8547, 109.0753)
  point P55 (-66.0346, 103.7753)
  point P56 (-75.8391, 101.8696)
  point P57 (-69.1332, 101.7373)
  point P58 (-77.6357, 95.4075)
  point P59 (-87.1527, 92.3765)
  point P60 (-80.4767, 93.0236)
  point P61 (-88.1869, 85.7494)
  point P62 (-97.2876, 81.634)
  point P63 (-90.7319, 83.0518)
  point P64 (-97.5455, 74.9317)
  point P65 (-106.107, 69.7876)
  point P66 (-99.7602, 71.9569)
  point P67 (-105.585, 63.1007)
  point P68 (-113.4913, 56.9975)
  point P69 (-107.4393, 59.8889)
  point P70 (-112.1966, 50.4164)
  point P71 (-119.341, 43.4366)
  point P72 (-113.6655, 47.011)
  point P73 (-117.2909, 37.0503)
  point P74 (-123.5767, 29.2882)
  point P75 (-118.3546, 33.4974)
  point P76 (-120.7991, 23.1831)
  point P77 (-126.1413, 14.7438)
  point P78 (-121.4431, 19.5307)
  point P79 (-122.6737, 9.0024)
  point P80 (-127, 0)
  point P81 (-122.8894, 5.3)
  point P82 (-122.8894, -5.3)
  point P83 (-126.1413, -14.7438)
  point P84 (-122.6737, -9.0024)
  point P85 (-121.4431, -19.5307)
  point P86 (-123.5767, -29.2882)
  point P87 (-120.7991, -23.1831)
  point P88 (-118.3546, -33.4974)
  point P89 (-119.341, -43.4366)
  point P90 (-117.2909, -37.0503)
  point P91 (-113.6655, -47.011)
  point P92 (-113.4913, -56.9975)
  point P93 (-112.1966, -50.4164)
  point P94 (-107.4393, -59.8889)
  point P95 (-106.107, -69.7876)
  point P96 (-105.585, -63.1007)
  point P97 (-99.7602, -71.9569)
  point P98 (-97.2876, -81.634)
  point P99 (-97.5455, -74.9317)
  point P100 (-90.7319, -83.0518)
  point P101 (-87.1527, -92.3765)
  point P102 (-88.1869, -85.7494)
  point P103 (-80.4767, -93.0236)
  point P104 (-75.8391, -101.8696)
  point P105 (-77.6357, -95.4075)
  point P106 (-69.1332, -101.7373)
  point P107 (-63.5, -109.9852)
  point P108 (-66.0346, -103.7753)
  point P109 (-56.8547, -109.0753)
  point P110 (-50.3021, -116.6134)
  point P111 (-53.5405, -110.7398)
  point P112 (-43.8074, -114.9382)
  point P113 (-36.424, -121.6647)
  point P114 (-40.3224, -116.2067)
  point P115 (-30.1677, -119.2468)
  point P116 (-22.0533, -125.0706)
  point P117 (-26.559, -120.1021)
  point P118 (-16.12, -121.9427)
  point P119 (-7.3844, -126.7851)
  point P120 (-12.4364, -122.3733)
  point P121 (-1.8543, -122.9896)
  point P122 (7.3844, -126.7851)
  point P123 (1.8543, -122.9896)
  point P124 (12.4364, -122.3733)
  point P125 (22.0533, -125.0706)
  point P126 (16.12, -121.9427)
  point P127 (26.559, -120.1021)
  point P128 (36.424, -121.6647)
  point P129 (30.1677, -119.2468)
  point P130 (40.3224, -116.2067)
  point P131 (50.3021, -116.6134)
  point P132 (43.8074, -114.9382)
  point P133 (53.5405, -110.7398)
  point P134 (63.5, -109.9852)
  point P135 (56.8547, -109.0753)
  point P136 (66.0346, -103.7753)
  point P137 (75.8391, -101.8696)
  point P138 (69.1332, -101.7373)
  point P139 (77.6357, -95.4075)
  point P140 (87.1527, -92.3765)
  point P141 (80.4767, -93.0236)
  point P142 (88.1869, -85.7494)
  point P143 (97.2876, -81.634)
  point P144 (90.7319, -83.0518)
  point P145 (97.5455, -74.9317)
  point P146 (106.107, -69.7876)
  point P147 (99.7602, -71.9569)
  point P148 (105.585, -63.1007)
  point P149 (113.4913, -56.9975)
  point P150 (107.4393, -59.8889)
  point P151 (112.1966, -50.4164)
  point P152 (119.341, -43.4366)
  point P153 (113.6655, -47.011)
  point P154 (117.2909, -37.0503)
  point P155 (123.5767, -29.2882)
  point P156 (118.3546, -33.4974)
  point P157 (120.7991, -23.1831)
  point P158 (126.1413, -14.7438)
  point P159 (121.4431, -19.5307)
  point P160 (122.6737, -9.0024)
  point P161 (94.9915, 58.7665)
  point P162 (103.1021, 74.1549)
  point P163 (91.5846, 63.9465)
  point P164 (87.5268, 69.397)
  point P165 (100.6097, 77.5029)
  point P166 (93.7961, 85.6229)
  point P167 (83.5416, 74.1465)
  point P168 (78.8785, 79.089)
  point P169 (83.2217, 95.9331)
  point P170 (74.3688, 83.3437)
  point P171 (69.1635, 87.7115)
  point P172 (71.5218, 104.9458)
  point P173 (64.1903, 91.4138)
  point P174 (58.5132, 95.1478)
  point P175 (58.8547, 112.5394)
  point P176 (53.1438, 98.2478)
  point P177 (47.0715, 101.2974)
  point P178 (55.1249, 114.4126)
  point P179 (45.3918, 118.6111)
  point P180 (41.3786, 103.7531)
  point P181 (34.9933, 106.0771)
  point P182 (31.3149, 123.0787)
  point P183 (29.0538, 107.8553)
  point P184 (22.4419, 109.4223)
  point P185 (16.8146, 125.882)
  point P186 (16.3361, 110.499)
  point P187 (9.587, 111.2878)
  point P188 (12.669, 126.3665)
  point P189 (2.0869, 126.9829)
  point P190 (3.3975, 111.6483)
  point P191 (-3.3975, 111.6483)
  point P192 (-2.0869, 126.9829)
  point P193 (-12.669, 126.3665)
  point P194 (-16.3361, 110.499)
  point P195 (-27.2536, 124.0413)
  point P196 (-22.4419, 109.4223)
  point P197 (-29.0538, 107.8553)
  point P198 (-41.4696, 120.0386)
  point P199 (-34.9933, 106.0771)
  dimension "d3" = 214.5
  dimension "d5" = 5.3
  dimension "d6" = 3.1
  dimension "d11" = 360
  constraints: 973 end point, 7 horizontal, 4 symmetric about line, 1 centre point, 1 coincident, 1350 other
  measures "d3" diameter of A0
  measures "d5" distance between parallel lines of L0 L3
  measures "d6" distance between parallel lines of L0 L2
extrude "Extrusion1" add sketch "Sketch1" along normal blind 34 contours A86 L5 L10 L7 A85 L4 L9 L2 | A2 A86 A3 A4 A5 A6 A7 A8 A9 A10 A11 A12 A13 A14 A15 A16 A17 A18 A19 A20 A21 A22 A23 A24 A25 A26 A27 A28 A29 A30 A31 A32 A33 A34 A35 A36 A37 A38 A39 A40 A41 A42 A43 A44 A45 A46 A47 A48 A49 A50 A51 A53 A52 A1 | L487 L485 L482 A85 L480 L484 L486 A86 | L478 L476 L473 A85 L471 L475 L477 A86 | A86 L19 L17 L14 A85 L12 L16 L18 | L469 L467 L464 A85 L462 L466 L468 A86 | A86 L28 L26 L23 A54 L21 L25 L27 | L460 L458 L455 A85 L453 L457 L459 A86 | A86 L37 L35 L32 A55 L30 L34 L36 | L451 L449 L446 A85 L444 L448 L450 A86 | A86 L46 L44 L41 A56 L39 L43 L45 | L442 L440 L437 A85 L435 L439 L441 A86 | A86 L55 L53 L50 A57 L48 L52 L54 | L433 L431 L428 A85 L426 L430 L432 A86 | A86 L64 L62 L59 A58 L57 L61 L63 | L424 L422 L419 A85 L417 L421 L423 A86 | A86 L73 L71 L68 A59 L66 L70 L72 | L415 L413 L410 A85 L408 L412 L414 A86 | A86 L82 L80 L77 A60 L75 L79 L81 | L406 L404 L401 A85 L399 L403 L405 A86 | A86 L91 L89 L86 A61 L84 L88 L90 | L397 L395 L392 A85 L390 L394 L396 A86 | A86 L100 L98 L95 A62 L93 L97 L99 | L388 L386 L383 A85 L381 L385 L387 A86 | A86 L109 L107 L104 A63 L102 L106 L108 | L379 L377 L374 A85 L372 L376 L378 A86 | A86 L118 L116 L113 A64 L111 L115 L117 | L370 L368 L365 A85 L363 L367 L369 A86 | A86 L127 L125 L122 A65 L120 L124 L126 | L361 L359 L356 A85 L354 L358 L360 A86 | A86 L136 L134 L131 A66 L129 L133 L135 | L352 L350 L347 A85 L345 L349 L351 A86 | A86 L145 L143 L140 A67 L138 L142 L144 | L343 L341 L338 A85 L336 L340 L342 A86 | A86 L154 L152 L149 A68 L147 L151 L153 | L334 L332 L329 A85 L327 L331 L333 A86 | A86 L163 L161 L158 A69 L156 L160 L162 | L325 L323 L320 A85 L318 L322 L324 A86 | A86 L172 L170 L167 A70 L165 L169 L171 | L316 L314 L311 A85 L309 L313 L315 A86 | A86 L181 L179 L176 A71 L174 L178 L180 | L307 L305 L302 A85 L300 L304 L306 A86 | A86 L190 L188 L185 A72 L183 L187 L189 | L298 L296 L293 A84 L291 L295 L297 A86 | A86 L199 L197 L194 A73 L192 L196 L198 | L289 L287 L284 A83 L282 L286 L288 A86 | A86 L208 L206 L203 A74 L201 L205 L207 | L280 L278 L275 A82 L273 L277 L279 A86 | A86 L217 L215 L212 A75 L210 L214 L216 | L271 L269 L266 A81 L264 L268 L270 A86 | A86 L226 L224 L221 A76 L219 L223 L225 | L262 L260 L257 A80 L255 L259 L261 A86 | A86 L235 L233 L230 A77 L228 L232 L234 | L253 L251 L248 A79 L246 L250 L252 A86 | A86 L244 L242 L239 A78 L237 L241 L243
body "Solid1"
